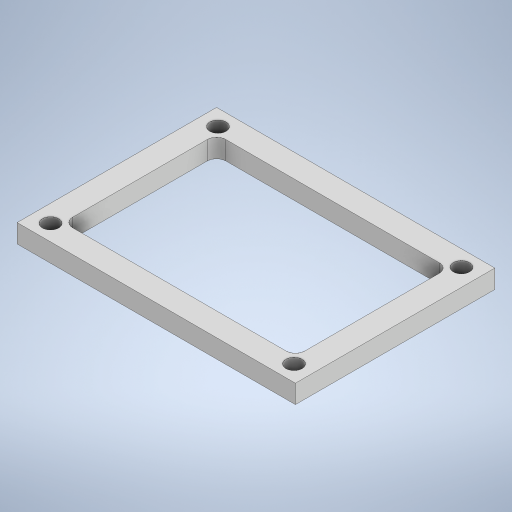
# Autodesk Inventor part: Buck 1
Saved by Autodesk Inventor 2024 (Build 280153000, 153)
## iProperties
Created: 2023-06-26
Part Number: Buck 1
Material: Genérico
Document SubType Name: Modeling
Designer: sergi
Density: 1 g/cm^3
Appearance: Valor por defecto
Author: sergi
Autodesk Inventor part; units mm, degrees
ref_plane "YZ Plane" through (0, 0, 0) normal (1, 0, 0) x (0, 1, 0)
ref_plane "XZ Plane" through (0, 0, 0) normal (0, 1, 0) x (-1, 0, 0)
ref_plane "XY Plane" through (0, 0, 0) normal (0, 0, 1) x (1, 0, 0)
sketch "Boceto1" plane through (0, 0, 0) normal (0, 1, 0) x (-1, 0, 0)
  line L0 (-30, -21.5) -> (30, -21.5)
  line L1 (30, -21.5) -> (30, 21.5)
  line L2 (30, 21.5) -> (-30, 21.5)
  line L3 (-30, 21.5) -> (-30, -21.5)
  line L4 (-30, -21.5) -> (30, 21.5) construction
  line L5 (30, -21.5) -> (-30, 21.5) construction
  line L6 (-23, 16.5) -> (23, 16.5)
  line L7 (25, 14.5) -> (25, -14.5)
  line L8 (23, -16.5) -> (-23, -16.5)
  line L9 (-25, -14.5) -> (-25, 14.5)
  line L10 (30, 21.5) -> (28, 21.5)
  line L11 (28, 21.5) -> (28, -21.5)
  line L12 (-30, 21.5) -> (-28, 21.5)
  line L13 (-28, 21.5) -> (-28, -21.5)
  line L14 (30, 21.5) -> (30, 19.8)
  line L15 (30, 19.8) -> (-30, 19.8)
  line L16 (30, -21.5) -> (30, -19.8)
  line L17 (30, -19.8) -> (-30, -19.8)
  circle A0 centre (26.25, -18.05) radius 1.75
  circle A1 centre (26.25, 18.05) radius 1.75
  circle A2 centre (-26.25, 18.05) radius 1.75
  circle A3 centre (-26.25, -18.05) radius 1.75
  arc A4 (25, 14.5) -> (23, 16.5) centre (23, 14.5) ccw
  arc A5 (23, -16.5) -> (25, -14.5) centre (23, -14.5) ccw
  arc A6 (-25, -14.5) -> (-23, -16.5) centre (-23, -14.5) ccw
  arc A7 (-23, 16.5) -> (-25, 14.5) centre (-23, 14.5) ccw
  point P0 (0, 0)
  dimension "d0" = 60
  dimension "d1" = 43
  dimension "d2" = 5
  dimension "d3" = 2
  dimension "d4" = 2
  dimension "d5" = 1.7
  dimension "d6" = 1.7
  dimension "d8" = 3.5
  dimension "d9" = 3.5
  dimension "d10" = 3.5
  dimension "d11" = 3.5
  dimension "d12" = 2
  dimension "d13" = 2
  constraints: 36 end point, 16 tangent, 8 centre point, 8 point on circle, 8 point on line, 5 parallel, 5 perpendicular, 2 equal radius, 2 midpoint, 1 horizontal, 3 other
  measures "d0" distance of L2.end L1.end
  measures "d1" distance of L1.end L0.end
  measures "d2" distance between parallel lines of L2 L6
  measures "d3" distance of L1.end L10.end
  measures "d4" distance of L2.end L12.end
  measures "d5" distance of L1.end L14.end
  measures "d6" distance of L0.end L16.end
  measures "d8" diameter of A0
  measures "d9" diameter of A1
  measures "d10" diameter of A2
  measures "d11" diameter of A3
  measures "d12" radius of A4
  measures "d13" radius of A5
extrude "Extrusión1" add sketch "Boceto1" along normal blind 4 contours L3 L17 L13 L0 | L13 L17 L11 L0 | L3 L15 L13 L17 | L11 L17 L1 L0 | L13 A3 L17 | L3 L2 L13 L15 | L17 A0 L11 | L11 L15 L1 L17 | L13 A2 L15 A1 L11 A0 L17 A3 | L15 A2 L13 | L13 L2 L11 L15 | L15 L11 L2 L1 | A1 L15 L11
